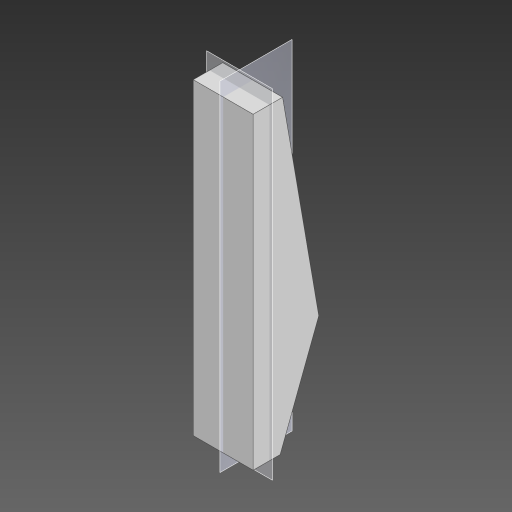
# Autodesk Inventor part: UpperArmBoundingBox
Saved by Autodesk Inventor 2023 (Build 270158000, 158)
## iProperties
Created: 2023-03-18
Part Number: UpperArmBoundingBox
Material: Generic
Document SubType Name: Modeling
Designer: Val
Density: 1 g/cm^3
Appearance: Default
Author: Val
Autodesk Inventor part; units mm, degrees
ref_plane "XZ Plane" through (0, 0, 0) normal (0, 1, 0) x (-1, 0, 0)
sketch "BoundingBox" plane through (0, 0, 0) normal (1, 0, 0) x (0, 1, 0)
  line L0 (434.8115, 24.0504) -> (-18, 24.0504)
  line L1 (-18, 24.0504) -> (-18, -15.6719)
  line L2 (-18, -15.6719) -> (130.2861, -72.3729)
  line L3 (130.2861, -72.3729) -> (434.8115, -19.2646)
  line L4 (434.8115, -19.2646) -> (434.8115, 24.0504)
  point P0 (0, 0)
  point P1 (417.3115, 0.6447)
  point P2 (-18, 4.1892)
  dimension "d5" = 24.0504
  dimension "d6" = 4.1893
  dimension "d7" = 110.926
  dimension "d8" = 452.8115
  dimension "d9" = 39.7223
  dimension "d10" = 43.315
  dimension "d11" = 99.893
  dimension "d12" = 56.7009
  dimension "d13" = 17.5
  dimension "d14" = 23.4057
  constraints: 10 end point, 2 perpendicular, 1 midpoint
  measures "d5" distance from line of L0 point (0, 0)
  measures "d6" vertical distance of point (-18, 4.189) point (0, 0)
  measures "d7" angle of L1 L2
  measures "d8" distance of L0.start L0.end
  measures "d9" distance of L0.end L1.end
  measures "d10" distance of L3.end L0.start
  measures "d11" angle of L4 L3
  measures "d12" vertical distance of L1.end L2.end
  measures "d13" distance from line of L4 point (417.312, 0.645)
  measures "d14" distance from line of L0 point (417.312, 0.645)
extrude "BoundingBoxFeature" add sketch "BoundingBox" along normal mid plane 88
body "Solid1"
